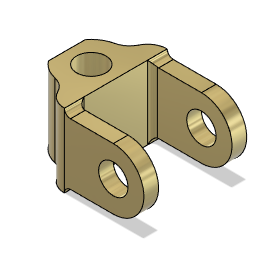
0.883.3687 - Croisillon à chape - VZC 21465_204997 (Autodesk Fusion 360 design; units mm, degrees)
Autodesk Fusion 360 part; units mm, degrees
sketch "Sketch1" plane through (0, 0, 0) normal (0, 0, 1) x (1, 0, 0)
  line L0 (0, 0) -> (50, 0) construction
  line L1 (0, 0) -> (0, 50) construction
  line L2 (0, 0) -> (-50, 0) construction
  line L3 (0, 0) -> (0, -50) construction
  line L4 (0, -15) -> (50, -15) construction
  line L5 (0, -15) -> (-50, -15) construction
  line L6 (0, 15) -> (-50, 15) construction
  line L7 (0, 15) -> (50, 15) construction
  line L8 (30, 0) -> (30, -50) construction
  line L9 (30, 0) -> (30, 50) construction
  line L10 (42.5, 0) -> (42.5, -50) construction
  line L11 (42.5, 0) -> (42.5, 50) construction
  line L12 (30, 12.5) -> (-12.5, 12.5)
  line L13 (30, -12.5) -> (-12.5, -12.5)
  arc A0 (30, -12.5) -> (30, 12.5) centre (30, 0) ccw
  line L14 (-12.5, 0) -> (-12.5, 50) construction
  line L15 (-12.5, 0) -> (-12.5, -50) construction
  line L16 (-12.5, 12.5) -> (-12.5, -12.5)
  line L17 (10, 0) -> (10, -50) construction
  line L18 (10, 0) -> (10, 50) construction
  line L19 (10, 12.5) -> (10, 15)
  line L20 (10, -12.5) -> (10, -15)
  line L21 (-12.5, -12.5) -> (-10, -15)
  line L22 (-12.5, -12.5) -> (-10, -12.5) construction
  line L23 (-10, -15) -> (10, -15)
  line L24 (-12.5, 12.5) -> (-10, 15)
  line L25 (-12.5, 12.5) -> (-2.5, 12.5) construction
  line L26 (-10, 15) -> (10, 15)
  circle A1 centre (30, 0) radius 6
  dimension "d5" = 15
  dimension "d6" = 15
  dimension "d7" = 30
  dimension "d8" = 42.5
  dimension "d9" = 12.5
  dimension "d10" = 10
  dimension "d11" = 45
  dimension "d14" = 45
  dimension "d15" = 12
  constraint coincident L0.start L1.start
  constraint horizontal L0
  constraint vertical L1
  constraint horizontal L2
  constraint vertical L3
  constraint coincident L8.start L9.start
  constraint coincident L10.start A0
  constraint tangent L11 A0
  constraint coincident L9 L12.start
  constraint tangent L12 A0
  constraint perpendicular L1 L12
  constraint coincident L8 L13.start
  constraint tangent L13 A0
  constraint perpendicular L3 L13
  constraint coincident L14 L12.end
  constraint perpendicular L13 L16
  constraint coincident L18 L19.start
  constraint coincident L12 L19.start
  constraint coincident L7 L19.end
  constraint coincident L18 L19.end
  constraint perpendicular L7 L19
  constraint coincident L17 L20.start
  constraint coincident L13 L20.start
  constraint coincident L4 L20.end
  constraint coincident L17 L20.end
  constraint perpendicular L4 L20
  constraint horizontal L22
  constraint perpendicular L17 L23
  constraint horizontal L25
  constraint coincident L6 L24.end
  constraint perpendicular L18 L26
  constraint concentric A0 A1
  measures "d11" angle of L21 L22
  measures "d14" angle of L24 L25
  measures "d15" diameter of A1
extrude "Extrude1" add sketch "Sketch1" along normal mid plane 42
sketch "Sketch2" plane through (0, 0, 0) normal (0, 1, 0) x (1, 0, 0)
  line L0 (30, -21) -> (42.5, -21) construction
  line L1 (42.5, 21) -> (30, 21) construction
  line L2 (10, 21) -> (30, 21) construction
  line L3 (30, -21) -> (10, -21) construction
  line L4 (10, -21) -> (-10, -21) construction
  line L5 (-10, -21) -> (-12.5, -21) construction
  line L6 (-12.5, -21) -> (-12.5, 21) construction
  line L7 (-10, 21) -> (10, 21) construction
  line L8 (-12.5, 21) -> (-10, 21) construction
  line L9 (42.5, -21) -> (42.5, 21) construction
  line L10 (42.5, -21) -> (42.5, -15) construction
  line L11 (42.5, 21) -> (42.5, 15) construction
  line L12 (42.5, -15) -> (12, -15)
  line L13 (42.5, 15) -> (12, 15)
  line L14 (10, -13) -> (10, 13)
  line L15 (42.5, -15) -> (42.5, 15)
  arc A0 (10, -13) -> (12, -15) centre (12, -13) ccw
  arc A1 (12, 15) -> (10, 13) centre (12, 13) ccw
  line L16 (0, 0) -> (-12.5, 0)
  line L17 (10, -21) -> (42.5, -21) construction
  line L18 (10, 21) -> (42.5, 21)
  line L19 (10, -21) -> (2, -21) construction
  line L20 (2, -21) -> (2, -13) construction
  line L21 (2, -13) -> (10, -13) construction
  line L22 (10, -13) -> (10, -21) construction
  arc A2 (2.8131, -16.514) -> (10, -21) centre (10, -13) ccw
  arc A3 (-12.5, 0) -> (-2.667, -12.2122) centre (0, 0) ccw
  arc A4 (2.8131, -16.514) -> (-2.667, -12.2122) centre (-4.3739, -20.028) ccw
  line L23 (-12.5, 0) -> (10, 0) construction
  arc A5 (-2.667, 12.2122) -> (-12.5, 0) centre (0, 0) ccw
  arc A6 (-2.667, 12.2122) -> (2.8131, 16.514) centre (-4.3739, 20.028) ccw
  arc A7 (10, 21) -> (2.8131, 16.514) centre (10, 13) ccw
  line L24 (10, -21) -> (-12.5, -21)
  line L25 (-12.5, -21) -> (-12.5, 21)
  line L26 (10, 21) -> (-12.5, 21)
  circle A8 centre (0, 0) radius 6
  point P0 (10, -15)
  point P1 (0, 15)
  dimension "d18" = 6
  dimension "d19" = 6
  dimension "d22" = 2
  dimension "d23" = 2
  dimension "d24" = 32.5
  dimension "d25" = 25
  dimension "d26" = 8
  dimension "d27" = 8
  dimension "d28" = 8
  dimension "d31" = 12
  constraint coincident L0.end L9.start
  constraint coincident L1.start L9.end
  constraint perpendicular L13 L14
  constraint perpendicular L13 L15
  constraint coincident P0 L12
  constraint coincident P0 L14
  constraint tangent L12 A0
  constraint tangent L14 A0
  constraint coincident P1 L13
  constraint tangent L13 A1
  constraint tangent L14 A1
  constraint coincident L16.start A3.centre
  constraint midpoint L6 L16.end
  constraint horizontal L12
  constraint coincident L3.end L4.start
  constraint perpendicular L10 L17
  constraint coincident L2.start L7.end
  constraint horizontal L19
  constraint vertical L20
  constraint horizontal L21
  constraint vertical L22
  constraint tangent A2 A4
  constraint tangent A3 A4
  constraint midpoint L14 L23.end
  constraint symmetric L16.end L23 A3.start
  constraint symmetric L3.end L23 L2.start
  constraint symmetric A2 L23 A7
  constraint symmetric A3 L23 A5
  constraint symmetric A2.start L23 A6.end
  constraint symmetric A3.end L23 A5.start
  constraint symmetric A4 L23 A6
  constraint coincident L5.end L6.start
  constraint tangent A2 L24
  constraint coincident L6.end L8.start
  measures "d18" distance of L0.end L10.end
  measures "d19" distance of L1.start L11.end
  measures "d22" radius of A0
  measures "d23" radius of A1
  measures "d24" distance of L9 L14
  measures "d25" diameter of A3
  measures "d26" distance of L3.end L19.end
  measures "d27" distance of L3.end L14.start
  measures "d28" radius of A4
  measures "d31" diameter of A8
extrude "Extrude2" cut sketch "Sketch2" along normal through all and the other way through all
fillet "Fillet1" radius 2.5 4 edges at (10, 12.5, 17) (10, 12.5, -17) (10, -12.5, -17) (10, -12.5, 17)
equation "d25 = ( 12.5 * 2 ) * 1 mm"
